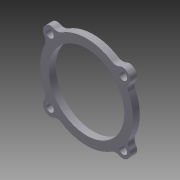
# Autodesk Inventor part: Cam.case.glassmount
Saved by Autodesk Inventor 2011 (Build 150239000, 239)
## iProperties
Created: 2011-03-23
Part Number: Cam.case.glassmount
Document SubType Name: Modeling
Designer: Rob
Density: 2.71 g/cm^3
Mass: 4.07021 g
Surface Area: 18.7489 cm^2
Volume: 1.50192 cm^3
Material: Aluminum-6061
Author: Rob
Autodesk Inventor part; units mm, degrees
note: some values were not read from the file. Chosen so that the rebuilt part matches the saved one: sketch regions of "Extrusion4".
ref_plane "YZ Plane" through (0, 0, 0) normal (1, 0, 0) x (0, 1, 0)
ref_plane "XZ Plane" through (0, 0, 0) normal (0, 1, 0) x (-1, 0, 0)
ref_plane "XY Plane" through (0, 0, 0) normal (0, 0, 1) x (1, 0, 0)
sketch "Sketch6" plane through (0, 0, 0) normal (0, 0, 1) x (1, 0, 0)
  circle A0 centre (3.9228, -14.5408) radius 10.15
  line L0 (10.903848, -34.81) -> (-10.903848, -34.81)
  line L1 (54.2, 8.803848) -> (54.2, -8.803848)
  circle A1 centre (3.9228, -14.5408) radius 16.4625
  circle A2 centre (19.9228, -0.5408) radius 1.5
  circle A3 centre (3.9228, -14.5408) radius 18.415
  line L2 (3.9228, -14.5408) -> (3.9228, -8.803848)
  line L3 (3.9228, -14.5408) -> (9.053444, -14.5408)
  circle A4 centre (3.9228, -14.5408) radius 20.2692
  line L4 (17.090037, 0.869078) -> (19.9228, 3.701841)
  line L5 (21.032601, -3.67364) -> (24.165441, -0.5408)
  line L6 (19.9228, 3.701841) -> (24.165441, -0.5408)
  line L7 (3.9228, -14.5408) -> (19.9228, -0.5408) construction
  line L8 (-12.0772, 3.701841) -> (-16.319841, -0.5408)
  line L9 (-13.187001, -3.67364) -> (-16.319841, -0.5408)
  circle A5 centre (-12.0772, -0.5408) radius 1.5
  line L10 (-9.244437, 0.869078) -> (-12.0772, 3.701841)
  line L11 (-9.244437, -29.950678) -> (-12.0772, -32.783441)
  line L12 (-12.0772, -32.783441) -> (-16.319841, -28.5408)
  circle A6 centre (-12.0772, -28.5408) radius 1.5
  line L13 (-13.187001, -25.40796) -> (-16.319841, -28.5408)
  line L14 (17.090037, -29.950678) -> (19.9228, -32.783441)
  line L15 (19.9228, -32.783441) -> (24.165441, -28.5408)
  line L16 (21.032601, -25.40796) -> (24.165441, -28.5408)
  circle A7 centre (19.9228, -28.5408) radius 1.5
  line L17 (24.165441, -28.5408) -> (18.258589, -22.633949)
  line L18 (19.9228, -32.783441) -> (14.388092, -27.248733)
  line L19 (-12.0772, -32.783441) -> (-6.542492, -27.248733)
  line L20 (-16.319841, -28.5408) -> (-10.412989, -22.633949)
  line L21 (-16.319841, -0.5408) -> (-10.412989, -6.447651)
  line L22 (-12.0772, 3.701841) -> (-6.542492, -1.832867)
  point P0 (0, 0)
  point P1 (0, 0)
  dimension "d53" = 32.925
  dimension "d54" = 3
  dimension "d55" = 36.83
  dimension "d56" = 14
  dimension "d57" = 16
  dimension "d58" = 45
  dimension "d59" = 3
  dimension "d60" = 3
  dimension "d61" = 3
  constraints: 46 end point, 15 symmetric about line, 8 centre point, 8 point on circle, 4 point on line, 3 coincident, 3 parallel, 3 perpendicular, 1 tangent, 3 other
  measures "d53" diameter of A1
  measures "d54" diameter of A2
  measures "d55" diameter of A3
  measures "d56" distance from line of L7.end L3
  measures "d57" distance from line of L2 L7.end
  measures "d58" angle of L2 L4
  measures "d59" distance from line of L4 L7.end
  measures "d60" distance from line of L5 L7.end
  measures "d61" distance from line of L7.end L6
extrude "Extrusion4" add sketch "Sketch6" along normal blind 3 contours A1 L22 A3 L17 | A1 L21 A3 L22 | L17 A3 L18 A1 | A1 L20 A3 L21 | L22 A4 A2 L17 A3 | A3 L21 A4 A5 L22 | L18 A3 L19 A1 | L17 A4 A7 L18 A3 | A1 L19 A3 L20 | A3 L20 A4 L21 | A4 A5 L9 L8 L10 | L18 A4 L19 A3 | L16 L15 L14 A4 A7 | A3 L19 A4 A6 L20 | L4 L6 L5 A4 A2 | A5 A4 | A4 A5 | A7 A4 | A4 A7 | A4 A6 L11 L12 L13 | A4 A2 | A2 A4 | A6 A4 | A4 A6
fillet "Fillet4" radius 3.5 8 edges at (-9.2444, 0.8691, 1.5) (-13.187, -3.6736, 1.5) (-13.187, -25.408, 1.5) (-9.2444, -29.9507, 1.5) (17.09, 0.8691, 1.5) (21.0326, -3.6736, 1.5) (21.0326, -25.408, 1.5) (17.09, -29.9507, 1.5)
fillet "Fillet5" radius 3 8 edges at (19.9228, 3.7018, 1.5) (24.1654, -0.5408, 1.5) (24.1654, -28.5408, 1.5) (19.9228, -32.7834, 1.5) (-16.3198, -28.5408, 1.5) (-12.0772, -32.7834, 1.5) (-16.3198, -0.5408, 1.5) (-12.0772, 3.7018, 1.5)
sketch "Sketch7" plane through (0, 0, 3) normal (0, 0, 1) x (1, 0, 0)
  circle A0 centre (3.9228, -14.5408) radius 10.15
  line L0 (10.903848, -34.81) -> (-10.903848, -34.81)
  line L1 (54.2, 8.803848) -> (54.2, -8.803848)
  circle A1 centre (3.9228, -14.5408) radius 16.4625
  circle A2 centre (19.9228, -0.5408) radius 1.5
  circle A3 centre (3.9228, -14.5408) radius 18.415
  line L2 (3.9228, -14.5408) -> (3.9228, -8.803848)
  line L3 (3.9228, -14.5408) -> (9.053444, -14.5408)
  circle A4 centre (3.9228, -14.5408) radius 20.2692
  line L4 (17.090037, 0.869078) -> (19.9228, 3.701841)
  line L5 (21.032601, -3.67364) -> (24.165441, -0.5408)
  line L6 (19.9228, 3.701841) -> (24.165441, -0.5408)
  line L7 (3.9228, -14.5408) -> (19.9228, -0.5408) construction
  line L8 (-12.0772, 3.701841) -> (-16.319841, -0.5408)
  line L9 (-13.187001, -3.67364) -> (-16.319841, -0.5408)
  circle A5 centre (-12.0772, -0.5408) radius 1.5
  line L10 (-9.244437, 0.869078) -> (-12.0772, 3.701841)
  line L11 (-9.244437, -29.950678) -> (-12.0772, -32.783441)
  line L12 (-12.0772, -32.783441) -> (-16.319841, -28.5408)
  circle A6 centre (-12.0772, -28.5408) radius 1.5
  line L13 (-13.187001, -25.40796) -> (-16.319841, -28.5408)
  line L14 (17.090037, -29.950678) -> (19.9228, -32.783441)
  line L15 (19.9228, -32.783441) -> (24.165441, -28.5408)
  line L16 (21.032601, -25.40796) -> (24.165441, -28.5408)
  circle A7 centre (19.9228, -28.5408) radius 1.5
  line L17 (24.165441, -28.5408) -> (18.258589, -22.633949)
  line L18 (19.9228, -32.783441) -> (14.388092, -27.248733)
  line L19 (-12.0772, -32.783441) -> (-6.542492, -27.248733)
  line L20 (-16.319841, -28.5408) -> (-10.412989, -22.633949)
  line L21 (-16.319841, -0.5408) -> (-10.412989, -6.447651)
  line L22 (-12.0772, 3.701841) -> (-6.542492, -1.832867)
  point P0 (0, 0)
  point P1 (0, 0)
  dimension "d66" = 32.925
  dimension "d67" = 3
  dimension "d68" = 36.83
  dimension "d69" = 14
  dimension "d70" = 16
  dimension "d71" = 45
  dimension "d72" = 3
  dimension "d73" = 3
  dimension "d74" = 3
  constraints: 46 end point, 15 symmetric about line, 8 centre point, 8 point on circle, 4 point on line, 3 coincident, 3 parallel, 3 perpendicular, 1 tangent, 3 other
  measures "d66" diameter of A1
  measures "d67" diameter of A2
  measures "d68" diameter of A3
  measures "d69" distance from line of L7.end L3
  measures "d70" distance from line of L2 L7.end
  measures "d71" angle of L2 L4
  measures "d72" distance from line of L4 L7.end
  measures "d73" distance from line of L5 L7.end
  measures "d74" distance from line of L7.end L6
hole "Hole3" at (-12.0772, -0.5408, 3) at (-12.0772, -28.5408, 3) at (19.9228, -28.5408, 3) at (19.9228, -0.5408, 3) direction (0, 0, -1) diameter 3.4036 depth 25.4 tip angle 118 clearance for "Flat Head Machine Screw" size "M3" standard "Ansi Metric M Profile"
body "Solid3"
